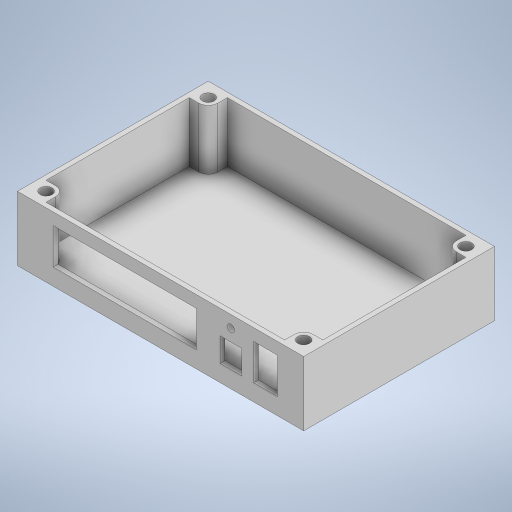
# Autodesk Inventor part: housing_base
Saved by Autodesk Inventor 2023 (Build 270158000, 158)
## iProperties
Created: 2023-05-09
Part Number: housing_base
Material: Generic
Document SubType Name: Modeling
Designer: mark
Density: 1 g/cm^3
Appearance: Default
Author: mark
Autodesk Inventor part; units mm, degrees
ref_plane "YZ Plane" through (0, 0, 0) normal (1, 0, 0) x (0, 1, 0)
ref_plane "XZ Plane" through (0, 0, 0) normal (0, 1, 0) x (-1, 0, 0)
ref_plane "XY Plane" through (0, 0, 0) normal (0, 0, 1) x (1, 0, 0)
sketch "Sketch1" plane through (0, 0, 0) normal (0, 1, 0) x (-1, 0, 0)
  line L0 (60, -40) -> (-60, -40)
  line L1 (-60, -40) -> (-60, 40)
  line L2 (-60, 40) -> (60, 40)
  line L3 (60, 40) -> (60, -40)
  point P0 (0, 0)
  dimension "d0" = 80
  dimension "d1" = 120
  dimension "d2" = 40
  dimension "d3" = 60
  constraints: 8 end point, 2 parallel, 1 horizontal, 1 perpendicular
  measures "d0" distance of L2.end L0.start
  measures "d1" distance of L0.start L0.end
  measures "d2" distance from line of point (0, 0) L0
  measures "d3" distance from line of point (0, 0) L3
extrude "Extrusion1" add sketch "Sketch1" along normal blind 2
sketch "Sketch2" plane through (0, 2, 0) normal (0, 1, 0) x (1, 0, 0)
  line L0 (60, 40) -> (-60, 40) projected
  line L1 (60, -40) -> (60, 40) projected
  line L2 (-60, 40) -> (60, 40)
  line L3 (60, 40) -> (60, -40)
  line L4 (60, -40) -> (-60, -40)
  line L5 (-60, -40) -> (-60, 40)
  line L6 (-58, 38) -> (58, 38)
  line L7 (58, 38) -> (58, -38)
  line L8 (58, -38) -> (-58, -38)
  line L9 (-58, -38) -> (-58, 38)
  arc A0 (-50, -34) -> (-54, -30) centre (-54, -34) ccw
  line L10 (-54, -30) -> (-58, -30)
  line L11 (-50, -34) -> (-50, -38)
  line L12 (0, 4.5233) -> (0, -3.3512)
  line L13 (-2.8256, 0) -> (3.7968, 0)
  arc A1 (-54, 30) -> (-50, 34) centre (-54, 34) ccw
  line L14 (-54, 30) -> (-58, 30)
  line L15 (-50, 34) -> (-50, 38)
  arc A2 (54, -30) -> (50, -34) centre (54, -34) ccw
  line L16 (54, -30) -> (58, -30)
  line L17 (50, -34) -> (50, -38)
  line L18 (54, 30) -> (58, 30)
  arc A3 (50, 34) -> (54, 30) centre (54, 34) ccw
  line L19 (50, 34) -> (50, 38)
  circle A4 centre (-54, -34) radius 2.5
  circle A5 centre (-54, 34) radius 2.5
  circle A6 centre (54, -34) radius 2.5
  circle A7 centre (54, 34) radius 2.5
  point P0 (0, 0)
  dimension "d6" = 2
  dimension "d7" = 2
  dimension "d8" = 2
  dimension "d9" = 2
  dimension "d29" = 8
  dimension "d30" = 4
  dimension "d31" = 4
  dimension "d32" = 5
  dimension "d35" = 68
  dimension "d38" = 108
  constraints: 36 end point, 15 symmetric about line, 8 centre point, 8 point on circle, 4 horizontal, 4 parallel, 4 perpendicular, 2 point on line, 2 tangent, 2 vertical, 1 coincident, 9 other
  measures "d6" distance between parallel lines of L0 L6
  measures "d7" distance between parallel lines of L5 L9
  measures "d8" distance between parallel lines of L4 L8
  measures "d9" distance between parallel lines of L1 L7
  measures "d29" diameter of A0
  measures "d30" distance from line of L9 A0.centre
  measures "d31" distance from line of L8 A0.centre
  measures "d32" diameter of A4
  measures "d35" distance of A4.centre A5.centre
  measures "d38" distance of A4.centre A6.centre
extrude "Extrusion2" add sketch "Sketch2" along normal blind 25 contours L1 L4 L5 L0 | L6 L15 A1 L14 L9 | L6 L7 L18 A3 L19 | L10 A0 L11 L8 L9 | L7 L8 L17 A2 L16
sketch "Sketch3" plane through (-60, 0, 40) normal (0, 0, 1) x (1, 0, 0)
  line L0 (15, 22) -> (75, 22)
  line L1 (75, 22) -> (75, 7)
  line L2 (75, 7) -> (15, 7)
  line L3 (15, 7) -> (15, 22)
  line L4 (10, 2) -> (110, 2) projected
  line L5 (0, 0) -> (0, 27) projected
  line L6 (85, 17) -> (94, 17)
  line L7 (94, 17) -> (94, 7)
  line L8 (94, 7) -> (85, 7)
  line L9 (85, 7) -> (85, 17)
  line L10 (99, 22) -> (109, 22)
  line L11 (109, 22) -> (109, 7)
  line L12 (109, 7) -> (99, 7)
  line L13 (99, 7) -> (99, 22)
  circle A0 centre (89.5, 22) radius 1.5
  point P0 (60, 0)
  point P1 (2, 2)
  point P2 (118, 2)
  point P3 (89.5, 7)
  point P4 (89.5, 17)
  dimension "d12" = 60
  dimension "d13" = 15
  dimension "d14" = 5
  dimension "d15" = 15
  dimension "d16" = 9
  dimension "d17" = 10
  dimension "d18" = 10
  dimension "d19" = 5
  dimension "d20" = 10
  dimension "d21" = 15
  dimension "d22" = 5
  dimension "d23" = 5
  dimension "d24" = 3
  dimension "d25" = 5
  dimension "d26" = 4.5
  constraints: 24 end point, 6 parallel, 3 horizontal, 3 perpendicular, 2 midpoint, 1 centre point
  measures "d12" distance of L0.start L0.end
  measures "d13" distance of L2.end L0.start
  measures "d14" distance between parallel lines of L4 L2
  measures "d15" distance between parallel lines of L5 L3
  measures "d16" distance of L7.end L8.end
  measures "d17" distance of L6.end L7.end
  measures "d18" distance between parallel lines of L1 L9
  measures "d19" distance from line of L4 point (89.5, 7)
  measures "d20" distance of L11.end L12.end
  measures "d21" distance of L10.end L11.end
  measures "d22" distance between parallel lines of L4 L12
  measures "d23" distance between parallel lines of L13 L7
  measures "d24" diameter of A0
  measures "d25" distance of point (89.5, 17) A0.centre
  measures "d26" distance from line of L9 A0.centre
extrude "Extrusion3" cut sketch "Sketch3" against normal blind 25
equation "\"d0\" = 0.666667 * d1"
equation "\"d2\" = 0.5 * d0"
equation "\"d3\" = 0.5 * d1"
equation "\"d7\" = d6"
equation "\"d8\" = d6"
equation "\"d9\" = d6"
equation "\"d30\" = 0.5 * d29"
equation "\"d31\" = d30"
equation "\"d19\" = d14"
equation "\"d22\" = d19"
equation "\"d26\" = 0.5 * d16"
body "Solid1"
